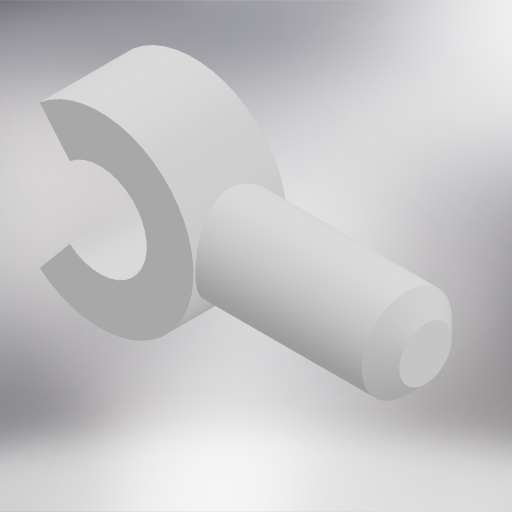
# Autodesk Inventor part: joint_part_black_2
Saved by Autodesk Inventor 2024 (Build 280153000, 153)
## iProperties
Created: 2023-10-25
Part Number: joint_part_black_2
Material: Generic
Document SubType Name: Modeling
Designer: SSAFY
Density: 1 g/cm^3
Appearance: Default
Author: SSAFY
Autodesk Inventor part; units mm, degrees
ref_plane "YZ Plane" through (0, 0, 0) normal (1, 0, 0) x (0, 1, 0)
ref_plane "XZ Plane" through (0, 0, 0) normal (0, 1, 0) x (-1, 0, 0)
ref_plane "XY Plane" through (0, 0, 0) normal (0, 0, 1) x (1, 0, 0)
sketch "Sketch1" plane through (0, 0, 0) normal (0, 0, 1) x (1, 0, 0)
  circle A0 centre (0, 0) radius 5
  circle A1 centre (0, 0) radius 2.5
  line L0 (0, 0) -> (-5, 0) construction
  line L1 (0, 0) -> (-3.2139, 3.8302)
  line L2 (0, 0) -> (-3.2139, -3.8302)
  line L3 (4.3863, 2.4) -> (14.3863, 2.4)
  line L4 (14.3863, 2.4) -> (14.3863, -2.4)
  line L5 (14.3863, -2.4) -> (4.3863, -2.4)
  line L6 (4.3863, -2.4) -> (4.3863, 2.4)
  point P0 (-1.607, 1.9151)
  point P1 (-1.607, -1.9151)
  dimension "d0" = 10
  dimension "d1" = 5
  dimension "d2" = 50
  dimension "d3" = 50
  dimension "d4" = 4.8
  dimension "d5" = 10
  constraints: 14 end point, 5 point on circle, 2 centre point, 2 coincident, 2 horizontal, 2 parallel, 1 perpendicular
  measures "d0" diameter of A0
  measures "d1" diameter of A1
  measures "d2" angle of L0 L1
  measures "d3" angle of L2 L0
  measures "d4" distance of L3.end L4.end
  measures "d5" distance of L3.start L3.end
extrude "Extrusion1" add sketch "Sketch1" along normal mid plane 5 contours A0 L6 | L6 A0 L2 A1 L1
sketch "Sketch2" plane through (0, 0, 0) normal (0, 0, 1) x (1, 0, 0)
  arc A0 (-3.2139, -3.8302) -> (-3.2139, 3.8302) centre (0, 0) ccw construction
  line L0 (4.3863, 2.4) -> (14.8863, 2.4)
  line L1 (14.8863, 2.4) -> (14.8863, -2.4)
  line L2 (14.8863, -2.4) -> (4.3863, -2.4)
  line L3 (4.3863, -2.4) -> (4.3863, 2.4)
  line L4 (4.3863, 0) -> (14.8863, 0)
  dimension "d8" = 4.8
  dimension "d9" = 10.5
  constraints: 10 end point, 2 midpoint, 2 parallel, 2 point on circle, 1 horizontal, 1 perpendicular
  measures "d8" distance of L0.end L1.end
  measures "d9" distance of L0.start L0.end
revolve "Revolution1" add sketch "Sketch2" angle 360 about axis through (4.3863, 0, 0) along (1, 0, 0) contours L0 L1 L4 L3
chamfer "Chamfer1" distance 1 angle 45 1 edges at (14.8863, -2.4, 0)
body "Solid1"
